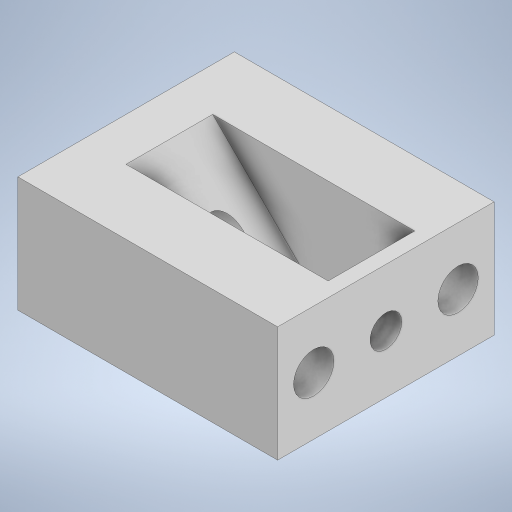
# Autodesk Inventor part: uchyceni_pruziny
Saved by Autodesk Inventor 2023.1 (Build 271208000, 208)
## iProperties
Created: 2023-01-12
Part Number: uchyceni_pruziny
Material: Všeobecné
Document SubType Name: Modeling
Designer: zavrel
Density: 1 g/cm^3
Appearance: Výchozí
Author: zavrel
Autodesk Inventor part; units mm, degrees
ref_plane "YZ Plane" through (0, 0, 0) normal (1, 0, 0) x (0, 1, 0)
ref_plane "XZ Plane" through (0, 0, 0) normal (0, 1, 0) x (-1, 0, 0)
sketch "Náčrt1" plane through (0, 0, 0) normal (0, 1, 0) x (-1, 0, 0)
  line L0 (0, 0) -> (0, -15)
  line L1 (0, -15) -> (18, -15)
  line L2 (18, -15) -> (18, 0)
  line L3 (18, 0) -> (0, 0)
  dimension "d0" = 15
  dimension "d1" = 18
  constraints: 8 end point, 3 perpendicular, 1 vertical
  measures "d0" distance of L0.start L0.end
  measures "d1" distance of L0.end L1.end
extrude "Vysunutí1" add sketch "Náčrt1" along normal blind 8
sketch "Náčrt2" plane through (0, 0, 0) normal (1, 0, 0) x (0, 0, -1)
  line L0 (0, 0) -> (15, 0) projected
  line L1 (15, 0) -> (15, 8) projected
  line L2 (0, 8) -> (15, 8) projected
  line L3 (0, 0) -> (0, 8) projected
  circle A0 centre (12.5, 4) radius 1.4
  line L4 (15, 8) -> (0, 8) projected
  line L5 (7.5, 8) -> (7.5, 0) construction
  circle A1 centre (2.5, 4) radius 1.4
  point P0 (15, 4)
  dimension "d4" = 10
  dimension "d7" = 2.8
  constraints: 3 midpoint, 2 centre point, 2 end point, 1 horizontal alignment, 1 symmetric about line, 1 other
  measures "d4" distance of A0.centre A1.centre
  measures "d7" diameter of A1
extrude "Vysunutí2" cut sketch "Náčrt2" against normal blind 10 contours A0 | A1
sketch "Náčrt3" plane through (-18, 0, -15) normal (-1, 0, 0) x (0, 0, 1)
  line L0 (0, 0) -> (15, 0) projected
  line L1 (15, 0) -> (15, 8) projected
  line L2 (0, 8) -> (15, 8) projected
  line L3 (0, 0) -> (0, 8) projected
  circle A0 centre (7.5, 4) radius 1.1
  point P0 (15, 0)
  dimension "d8" = 2.2
  constraints: 1 centre point
  measures "d8" diameter of A0
extrude "Vysunutí3" cut sketch "Náčrt3" against normal through all contours A0
ref_plane "Pracovní rovina1" through (0, 0, -7.5) normal (0, 0, -1) x (-1, 0, 0)
sketch "Náčrt4" plane through (0, 0, -7.5) normal (0, 0, -1) x (-1, 0, 0)
  line L0 (0, 0) -> (18, 0) projected
  line L1 (18, 0) -> (18, 8) projected
  line L2 (0, 8) -> (18, 8) projected
  line L3 (0, 0) -> (0, 8) projected
  line L4 (1, 8) -> (8, 1)
  line L5 (8, 1) -> (15, 8)
  point P0 (0, 0)
  dimension "d11" = 90
  dimension "d12" = 7
  dimension "d15" = 8
  constraints: 4 end point, 2 point on line, 1 perpendicular
  measures "d11" angle of L4 L5
  measures "d12" distance from line of L4.end L2
  measures "d15" distance from line of L3 L4.end
extrude "Vysunutí4" cut sketch "Náčrt4" along normal mid plane 6 contours L2 L5 L4
